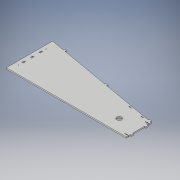
# Autodesk Inventor part: pinball-case-left-wall
Saved by Autodesk Inventor 2017 (Build 210142000, 142)
## iProperties
Created: 2017-02-27
Part Number: pinball-case-left-wall
Material: Generic
Document SubType Name: Modeling
Designer: John
Density: 1 g/cm^3
Appearance: Default
Author: John
Autodesk Inventor part; units mm, degrees
ref_plane "YZ Plane" through (0, 0, 0) normal (1, 0, 0) x (0, 1, 0)
ref_plane "XZ Plane" through (0, 0, 0) normal (0, 1, 0) x (-1, 0, 0)
ref_plane "XY Plane" through (0, 0, 0) normal (0, 0, 1) x (1, 0, 0)
sketch "Sketch1" plane through (0, 0, 0) normal (0, 1, 0) x (-1, 0, 0)
  line L0 (0, 0) -> (-590, 0)
  line L1 (-590, 0) -> (-590, -120.9671)
  line L2 (-590, -120.9671) -> (0, -120.9671)
  line L3 (0, -120.9671) -> (0, 0)
  line L4 (0, -120.9671) -> (0, -225)
  line L5 (0, -225) -> (-590, -120.9671)
  dimension "d0" = 590
  dimension "d50" = 225
  dimension "d51" = 10
  constraints: 12 end point, 2 parallel, 1 horizontal, 1 perpendicular, 1 vertical
  measures "d0" distance of L2.end L1.end
  measures "d50" distance of L0.start L4.end
  measures "d51" angle of L2 L5
extrude "Extrusion1" add sketch "Sketch1" along normal blind 6
sketch "Sketch2" plane through (0, 6, 0) normal (0, 1, 0) x (1, 0, 0)
  line L0 (62.143, 214.0425) -> (73.9607, 211.9587)
  line L1 (73.9607, 211.9587) -> (75.0026, 217.8676)
  line L2 (75.0026, 217.8676) -> (63.1849, 219.9514)
  line L3 (63.1849, 219.9514) -> (62.143, 214.0425)
  line L4 (0, 225) -> (62.143, 214.0425) construction
  line L5 (590, 120.9671) -> (578.1823, 123.0509) construction
  line L6 (590, 120.9671) -> (0, 225) construction
  line L7 (578.1823, 123.0509) -> (566.3646, 125.1346)
  line L8 (566.3646, 125.1346) -> (567.4065, 131.0435)
  line L9 (567.4065, 131.0435) -> (579.2242, 128.9597)
  line L10 (579.2242, 128.9597) -> (578.1823, 123.0509)
  line L11 (320.1627, 168.5467) -> (308.345, 170.6305)
  line L12 (308.345, 170.6305) -> (309.3869, 176.5393)
  line L13 (309.3869, 176.5393) -> (321.2046, 174.4555)
  line L14 (321.2046, 174.4555) -> (320.1627, 168.5467)
  point P0 (0, 0)
  dimension "d5" = 6
  dimension "d7" = 12
  dimension "d9" = 12
  dimension "d10" = 12
  dimension "d11" = 6
  dimension "d14" = 500
  dimension "d15" = 12
  dimension "d16" = 6
  dimension "d17" = 250
  constraints: 28 end point, 6 parallel, 3 perpendicular, 3 point on line, 1 collinear
  measures "d5" distance of L1.end L0.end
  measures "d7" distance between parallel lines of L1 L3
  measures "d9" distance of L5.start L5.end
  measures "d10" distance of L5.end L7.end
  measures "d11" distance of L7.end L8.end
  measures "d14" distance between parallel lines of L8 L1
  measures "d15" distance of L11.start L11.end
  measures "d16" distance of L11.end L12.end
  measures "d17" distance between parallel lines of L14 L8
extrude "Extrusion2" add sketch "Sketch2" against normal blind 6
sketch "Sketch3" plane through (0, 6, 0) normal (0, 1, 0) x (1, 0, 0)
  line L0 (590, 0) -> (590, 120.9671) projected
  line L1 (590, 126) -> (584, 126)
  line L2 (584, 126) -> (584, 101)
  line L3 (584, 101) -> (590, 101)
  line L4 (590, 101) -> (590, 126)
  line L5 (590, 0) -> (584, 0)
  line L6 (584, 0) -> (584, 20)
  line L7 (584, 20) -> (590, 20)
  line L8 (590, 20) -> (590, 0)
  line L9 (590, 89) -> (584, 89)
  line L10 (584, 89) -> (584, 32)
  line L11 (584, 32) -> (590, 32)
  line L12 (590, 32) -> (590, 89)
  point P0 (0, 0)
  dimension "d18" = 6
  dimension "d20" = 6
  dimension "d21" = 20
  dimension "d22" = 12
  dimension "d23" = 12
  dimension "d27" = 57
  dimension "d36" = 25
  constraints: 24 end point, 6 parallel, 3 horizontal, 3 perpendicular, 1 point on line
  measures "d18" distance of L3.end L2.end
  measures "d20" distance of L6.end L7.end
  measures "d21" distance of L5.end L6.end
  measures "d22" distance between parallel lines of L3 L9
  measures "d23" distance between parallel lines of L7 L11
  measures "d27" distance of L9.end L10.end
  measures "d36" distance of L1.end L2.end
extrude "Extrusion3" cut sketch "Sketch3" along normal through all both and the other way through all
sketch "Sketch4" plane through (0, 6, 0) normal (0, 1, 0) x (1, 0, 0)
  line L0 (584, 0) -> (584, 20) projected
  line L1 (584, 12) -> (576, 12)
  line L2 (567, 12) -> (567, 9.5)
  line L3 (567, 9.5) -> (573.7, 9.5)
  line L4 (584, 9.5) -> (584, 12)
  line L5 (0, 0) -> (584, 0) construction
  line L6 (573.7, 13.45) -> (576, 13.45)
  line L7 (576, 13.45) -> (576, 12)
  line L8 (576, 8.05) -> (573.7, 8.05)
  line L9 (573.7, 8.05) -> (573.7, 9.5)
  line L10 (576, 12) -> (576, 9.5) construction
  line L11 (576, 9.5) -> (576, 8.05)
  line L12 (573.7, 12) -> (573.7, 13.45)
  line L13 (573.7, 9.5) -> (573.7, 12) construction
  line L14 (576, 12) -> (573.7, 12) construction
  line L15 (573.7, 12) -> (567, 12)
  line L16 (576, 9.5) -> (584, 9.5)
  line L17 (573.7, 9.5) -> (576, 9.5) construction
  line L18 (584, 111.5) -> (576, 111.5)
  line L19 (567, 111.5) -> (567, 109)
  line L20 (567, 109) -> (573.7, 109)
  line L21 (584, 109) -> (584, 111.5)
  line L22 (573.7, 112.95) -> (576, 112.95)
  line L23 (576, 112.95) -> (576, 111.5)
  line L24 (576, 107.55) -> (573.7, 107.55)
  line L25 (573.7, 107.55) -> (573.7, 109)
  line L26 (576, 111.5) -> (576, 109) construction
  line L27 (576, 109) -> (576, 107.55)
  line L28 (573.7, 111.5) -> (573.7, 112.95)
  line L29 (573.7, 109) -> (573.7, 111.5) construction
  line L30 (576, 111.5) -> (573.7, 111.5) construction
  line L31 (573.7, 111.5) -> (567, 111.5)
  line L32 (576, 109) -> (584, 109)
  line L33 (573.7, 109) -> (576, 109) construction
  line L34 (590, 101) -> (584, 101) construction
  line L35 (584, 20) -> (590, 20) construction
  line L36 (14.1705, 156) -> (20.1705, 156)
  line L37 (20.1705, 156) -> (20.1705, 144)
  line L38 (20.1705, 144) -> (14.1705, 144)
  line L39 (14.1705, 144) -> (14.1705, 156)
  line L40 (15, 114) -> (21, 114)
  line L41 (21, 114) -> (21, 102)
  line L42 (21, 102) -> (15, 102)
  line L43 (15, 102) -> (15, 114)
  line L44 (15, 72) -> (21, 72)
  line L45 (21, 72) -> (21, 60)
  line L46 (21, 60) -> (15, 60)
  line L47 (15, 60) -> (15, 72)
  line L48 (0, 225) -> (0, 0) projected
  circle A0 centre (17.1705, 176) radius 1.25
  circle A1 centre (18, 40) radius 1.25
  line L49 (18, 60) -> (18, 40) construction
  point P0 (584, 122.025)
  dimension "d37" = 17
  dimension "d38" = 2.5
  dimension "d58" = 2.3
  dimension "d59" = 5.4
  dimension "d60" = 8
  dimension "d66" = 17
  dimension "d67" = 2.5
  dimension "d68" = 2.3
  dimension "d69" = 5.4
  dimension "d70" = 8
  dimension "d71" = 8
  dimension "d72" = 6
  dimension "d73" = 12
  dimension "d77" = 30
  dimension "d78" = 30
  dimension "d79" = 60
  dimension "d80" = 15
  dimension "d81" = 2.5
  dimension "d82" = 2.5
  dimension "d83" = 20
  dimension "d84" = 20
  constraints: 90 end point, 46 parallel, 15 perpendicular, 11 horizontal, 5 equal length, 5 point on line, 2 centre point, 1 midpoint, 1 vertical
  measures "d37" distance of L4.start L2.end
  measures "d38" distance of L2.end L2.start
  measures "d58" distance of L8.start L8.end
  measures "d59" distance of L6.end L8.start
  measures "d60" distance between parallel lines of L0 L7
  measures "d66" distance of L21.start L19.end
  measures "d67" distance of L19.end L31.end
  measures "d68" distance of L24.start L24.end
  measures "d69" distance of L22.end L24.start
  measures "d70" distance between parallel lines of L34 L32
  measures "d71" distance between parallel lines of L1 L35
  measures "d72" distance of L37.end L38.end
  measures "d73" distance of L36.end L37.end
  measures "d77" distance between parallel lines of L38 L40
  measures "d78" distance between parallel lines of L44 L42
  measures "d79" distance between parallel lines of L46 L5
  measures "d80" distance between parallel lines of L48 L47
  measures "d81" diameter of A0
  measures "d82" diameter of A1
  measures "d83" distance from line of L49.end L46
  measures "d84" distance from line of L36 A0.centre
extrude "Extrusion4" cut sketch "Sketch4" along normal through all both and the other way through all
sketch "Sketch5" plane through (0, 6, 0) normal (0, 1, 0) x (1, 0, 0)
  circle A0 centre (490, 60) radius 12
  line L0 (0, 0) -> (584, 0) projected
  line L1 (590, 89) -> (590, 101) projected
  dimension "d45" = 24
  dimension "d46" = 60
  dimension "d47" = 100
  constraints: 1 centre point
  measures "d45" diameter of A0
  measures "d46" distance from line of L0 A0.centre
  measures "d47" distance from line of L1 A0.centre
extrude "Extrusion5" cut sketch "Sketch5" against normal through all
sketch "Sketch6" plane through (0, 6, 0) normal (0, 1, 0) x (1, 0, 0)
  line L0 (533.8089, 124.7825) -> (545.6266, 122.6988)
  line L1 (545.6266, 122.6988) -> (545.1056, 119.7443)
  line L2 (545.1056, 119.7443) -> (533.2879, 121.8281)
  line L3 (533.2879, 121.8281) -> (533.8089, 124.7825)
  line L4 (474.7204, 135.2014) -> (462.9027, 137.2852)
  line L5 (462.9027, 137.2852) -> (462.3818, 134.3308)
  line L6 (462.3818, 134.3308) -> (474.1995, 132.247)
  line L7 (474.1995, 132.247) -> (474.7204, 135.2014)
  line L8 (566.3646, 125.1346) -> (320.1627, 168.5467) projected
  point P0 (0, 0)
  dimension "d85" = 12
  dimension "d86" = 3
  dimension "d87" = 12
  dimension "d88" = 60
  dimension "d89" = 20
  dimension "d92" = 6
  constraints: 16 end point, 5 parallel, 2 perpendicular, 2 point on line, 1 collinear
  measures "d85" distance of L1.end L2.end
  measures "d86" distance of L0.end L1.end
  measures "d87" distance of L6.end L5.end
  measures "d88" distance between parallel lines of L7 L3
  measures "d89" distance from line of L1 L8.start
  measures "d92" distance between parallel lines of L0 L8
extrude "Extrusion6" cut sketch "Sketch6" against normal through all
equation "\"d18\" = d20"
equation "\"d23\" = d22"
equation "\"d78\" = d77"
equation "\"d81\" = d82"
equation "\"d84\" = d83"
body "Solid1"
